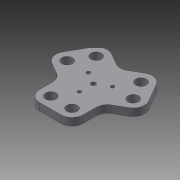
# Autodesk Inventor part: Effector_Platform_V2
Saved by Autodesk Inventor 2014 (Build 180170000, 170)
## iProperties
Created: 2014-10-18
Part Number: Effector_Platform_V2
Material: Generic
Document SubType Name: Modeling
Designer: ThatOtherGuy
Density: 1 g/cm^3
Appearance: Default
Author: ThatOtherGuy
Autodesk Inventor part; units mm, degrees
note: some values were not read from the file. Chosen so that the rebuilt part matches the saved one: edges of "Fillet1".
ref_plane "YZ Plane" through (0, 0, 0) normal (1, 0, 0) x (0, 1, 0)
ref_plane "XZ Plane" through (0, 0, 0) normal (0, 1, 0) x (-1, 0, 0)
ref_plane "XY Plane" through (0, 0, 0) normal (0, 0, 1) x (1, 0, 0)
sketch "Sketch1" plane through (0, 0, 0) normal (0, 0, 1) x (1, 0, 0)
  line L0 (0, 0) -> (-33.403, 19.2853)
  line L1 (0, 0) -> (33.403, 19.2853)
  arc A0 (1.8187, 1.05) -> (-1.8187, 1.05) centre (0, 0) ccw
  circle A1 centre (-20, 22.5) radius 4.75
  circle A2 centre (20, 22.5) radius 4.75
  line L2 (0, 0) -> (-27.7881, 0)
  line L3 (-33.403, 19.2853) -> (-23.6603, 36.1603)
  line L4 (23.6603, 36.1603) -> (33.403, 19.2853)
  line L5 (-23.6603, 36.1603) -> (0, 22.5)
  line L6 (0, 22.5) -> (23.6603, 36.1603)
  dimension "d0" = 120
  dimension "d1" = 2.1
  dimension "d2" = 9.5
  dimension "d3" = 40
  dimension "d4" = 20
  dimension "d5" = 22.5
  dimension "d6" = 30
  dimension "d10" = 10
  dimension "d30" = 10
  constraints: 14 end point, 3 centre point, 3 perpendicular, 2 equal length, 2 point on circle, 2 point on line, 1 coincident, 1 equal radius, 1 horizontal, 1 horizontal alignment, 1 parallel
  measures "d0" angle of L1 L0
  measures "d1" radius of A0
  measures "d2" diameter of A2
  measures "d3" distance of A2.centre A1.centre
  measures "d4" horizontal distance of L0.start A1.centre
  measures "d5" vertical distance of L0.start A1.centre
  measures "d6" angle of L0 L2
  measures "d10" distance from line of L3 A1.centre
  measures "d30" distance from line of L5 A1.centre
extrude "Extrusion1" add sketch "Sketch1" along normal blind 6.731 contours L0 L3 L5 L6 L4 L1 A0
fillet "Fillet1" radius 10 3 edges at (-23.6603, 36.1603, 3.3655) (23.6603, 36.1603, 3.3655) (0, 22.5, 3.3655)
pattern_circular "Circular Pattern1" count 3 over 360 about axis through (0, 0, 0) along (0, 0, 1) of "Extrusion1", "Fillet1"
sketch "Sketch2" plane through (0, 0, 0) normal (0, 0, -1) x (-1, 0, 0)
  circle A0 centre (0, 0) radius 2.1 projected
  circle A1 centre (10.8253, 6.25) radius 1.6
  line L0 (19.4856, -17.0235) -> (19.4856, -28.5705) projected
  line L1 (10.8253, 6.25) -> (0, 0) construction
  line L2 (0, 0) -> (15.25, 0) construction
  point P0 (19.4856, -18.9295)
  dimension "d18" = 3.2
  dimension "d20" = 12.5
  dimension "d33" = 30
  constraints: 4 end point, 1 centre point, 1 perpendicular
  measures "d18" diameter of A1
  measures "d20" distance of L1.end L1.start
  measures "d33" angle of L2 L1
extrude "Extrusion2" cut sketch "Sketch2" against normal up to next contours A1
pattern_circular "Circular Pattern2" count 3 over 360 about axis through (0, 0, 0) along (0, 0, 1) of "Extrusion2"
sketch "Sketch3" plane through (0, 0, 0) normal (0, 0, -1) x (-1, 0, 0)
  circle A0 centre (0, 0) radius 2.1 projected
  circle A1 centre (0, 0) radius 8
  dimension "d26" = 16
  constraints: 1 centre point, 1 coincident
  measures "d26" diameter of A1
extrude "Extrusion3" cut sketch "Sketch3" against normal blind 3.6
equation "\"d2\" = MAGDIA"
equation "\"d4\" = 0.5 * d3"
equation "\"d30\" = d10"
equation "\"d12\" = THICKB"
equation "\"d21\" = THICKB"
equation "\"THICKA\" = 3.175"
equation "\"THICKB\" = 6.731"
equation "\"THICKC\" = 12.7"
equation "\"MAGDIA\" = 9.5"
equation "\"BALLDIA\" = 12"
equation "\"THICKPLY\" = 5"
body "Solid1"
